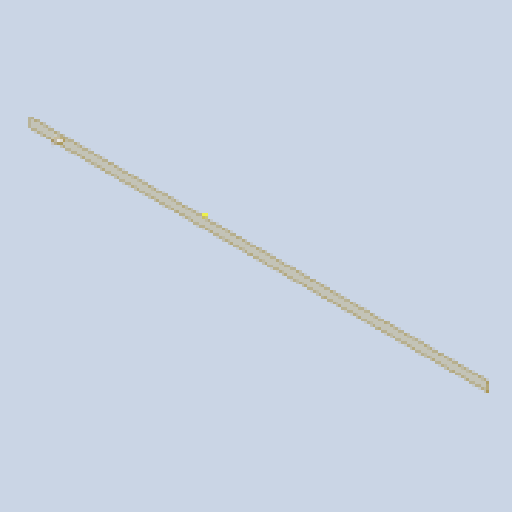
# Autodesk Inventor part: деталь крепление энкодера
Saved by Autodesk Inventor 2024.2 (Build 282272000, 272)
## iProperties
Created: 2025-12-24
Part Number: деталь крепление энкодера
Material: Типовые
Document SubType Name: Modeling
Designer: katya_notebook
Density: 1 g/cm^3
Appearance: По умолчанию
Author: katya_notebook
Autodesk Inventor part; units mm, degrees
ref_plane "YZ Plane" through (0, 0, 0) normal (1, 0, 0) x (0, 1, 0)
ref_plane "XZ Plane" through (0, 0, 0) normal (0, 1, 0) x (-1, 0, 0)
ref_plane "XY Plane" through (0, 0, 0) normal (0, 0, 1) x (1, 0, 0)
ref_plane "РабПлоскость2" through (-682.985, -17.9529, 102.0837) normal (0, 1, 0) x (-1, 0, 0)
ref_plane "РабПлоскость3" through (1272.2614, -51.4529, 81.5837) normal (0, 0, 1) x (1, 0, 0)
sketch "Эскиз1" plane through (1272.2614, -51.4529, 81.5837) normal (0, 0, 1) x (1, 0, 0)
  point P0 (-1272.2614, 51.4529)
sketch "Эскиз2" plane through (-682.985, -17.9529, 102.0837) normal (0, 1, 0) x (-1, 0, 0)
  line L0 (-11.5, -11.5) -> (11.5, -11.5)
  line L1 (11.5, -11.5) -> (11.5, 11.5)
  line L2 (11.5, 11.5) -> (-11.5, 11.5)
  line L3 (-11.5, 11.5) -> (-11.5, -11.5)
  line L4 (-11.5, -11.5) -> (11.5, 11.5) construction
  line L5 (11.5, -11.5) -> (-11.5, 11.5) construction
  circle A0 centre (8.5, 8.5) radius 2
  circle A1 centre (8.5, -8.5) radius 2
  line L6 (0, 20.5912) -> (0, -22.1181)
  circle A2 centre (-8.5, 8.5) radius 2
  circle A3 centre (-8.5, -8.5) radius 2
  point P0 (-682.985, -102.0837)
  point P1 (0, 0)
  point P2 (0, 0)
  dimension "d0" = 23
  dimension "d1" = 23
  dimension "d2" = 4
  dimension "d5" = 3
  dimension "d6" = 3
  dimension "d7" = 4
  dimension "d8" = 3
  dimension "d9" = 3
  constraints: 14 end point, 4 centre point, 2 midpoint, 2 parallel, 2 symmetric about line, 1 coincident, 1 horizontal, 1 perpendicular, 1 vertical, 3 other
  measures "d0" distance of L0.end L1.end
  measures "d1" distance of L1.end L2.end
  measures "d2" diameter of A0
  measures "d5" distance from line of L1 A0.centre
  measures "d6" distance from line of L2 A0.centre
  measures "d7" diameter of A1
  measures "d8" distance from line of L1 A1.centre
  measures "d9" distance from line of L0 A1.centre
extrude "Выдавливание1" add sketch "Эскиз2" along normal blind 2
sketch "Эскиз3" plane through (-694.485, -17.9529, 90.5837) normal (-1, 0, 0) x (0, 0, 1)
  line L0 (23, 0) -> (0, 0) projected
  line L1 (23, 2) -> (0, 2)
  line L2 (0, 2) -> (0, 0)
  line L3 (0, 0) -> (23, 0)
  line L4 (23, 0) -> (23, 2)
  point P0 (-90.5837, 17.9529)
  constraints: 8 end point, 2 parallel, 1 horizontal, 1 perpendicular
extrude "Выдавливание2" add sketch "Эскиз3" along normal blind 12
sketch "Эскиз6" plane through (-706.485, -17.9529, 90.5837) normal (-1, 0, 0) x (0, 0, 1)
  line L0 (23, 2) -> (0, 2)
  line L1 (0, 2) -> (0, -31.5)
  line L2 (0, -31.5) -> (23, -31.5)
  line L3 (23, -31.5) -> (23, 2)
  point P0 (-90.5837, 17.9529)
  dimension "d14" = 33.5
  constraints: 8 end point, 2 parallel, 1 horizontal, 1 perpendicular
  measures "d14" distance of L0.end L1.end
extrude "Выдавливание3" add sketch "Эскиз6" along normal blind 2
sketch "Эскиз7" plane through (-671.485, -17.9529, 113.5837) normal (1, 0, 0) x (0, 0, -1)
  point P0 (113.5837, 17.9529)
sketch "Эскиз8" plane through (-682.985, -17.9529, 102.0837) normal (0, 1, 0) x (-1, 0, 0)
  point P0 (-682.985, -102.0837)
sketch "Эскиз9" plane through (-671.485, -17.9529, 113.5837) normal (1, 0, 0) x (0, 0, -1)
  line L0 (23, 0) -> (23, 2) projected
  line L1 (23, 2) -> (0, 2)
  line L2 (0, 2) -> (0, 0)
  line L3 (0, 0) -> (23, 0)
  line L4 (23, 0) -> (23, 2)
  point P0 (113.5837, 17.9529)
  constraints: 8 end point, 2 parallel, 1 horizontal, 1 perpendicular
extrude "Выдавливание4" add sketch "Эскиз9" along normal blind 12
sketch "Эскиз10" plane through (-659.485, -17.9529, 113.5837) normal (1, 0, 0) x (0, 0, -1)
  line L0 (0, 2) -> (23, 2) projected
  line L1 (23, -31.5) -> (0, -31.5) projected
  line L2 (23, 2) -> (0, 2)
  line L3 (0, 2) -> (0, -31.5)
  line L4 (0, -31.5) -> (23, -31.5)
  line L5 (23, -31.5) -> (23, 2)
  point P0 (113.5837, 17.9529)
  point P1 (23, -31.5)
  constraints: 8 end point, 2 parallel, 1 horizontal, 1 perpendicular
extrude "Выдавливание5" add sketch "Эскиз10" along normal blind 2
